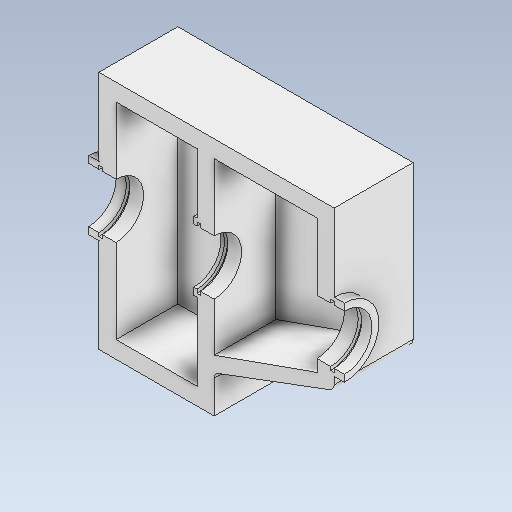
# Autodesk Inventor part: zmotorblockleft-half
Saved by Autodesk Inventor 2020 (Build 240168000, 168)
## iProperties
Created: 2020-11-21
Part Number: zmotorblockleft-half
Material: ABS Plastic
Document SubType Name: Modeling
Designer: AOB
Mass: 48.551 g
Surface Area: 203.359 cm^2
Volume: 45.8029 cm^3
Density: 1.06 g/cm^3
Appearance: Smooth - White
Author: AOB
Autodesk Inventor part; units mm, degrees
ref_plane "YZ Plane" through (0, 0, 0) normal (1, 0, 0) x (0, 1, 0)
sketch "Sketch1" plane through (0, 0, 0) normal (0, 0, 1) x (1, 0, 0)
  line L0 (16.1624, 3.9921) -> (16.1624, 53.6188)
  line L1 (16.0624, -11.3812) -> (-17.438, -11.3812)
  line L2 (-17.438, 58.6188) -> (48.5624, 58.6188)
  line L3 (-17.438, 58.6188) -> (-17.438, -11.3812)
  line L4 (-12.438, 53.6188) -> (-12.438, -6.3812)
  line L5 (11.1624, 53.6188) -> (11.1624, -6.3812)
  line L6 (43.5624, 53.6188) -> (46.1624, 53.6188)
  line L7 (11.1624, 53.6188) -> (-12.438, 53.6188)
  line L8 (-12.438, -6.3812) -> (11.1624, -6.3812)
  line L9 (18.7626, 0.4857) -> (43.5624, 9.7508)
  line L10 (16.1624, -1.8735) -> (16.1624, -11.3812)
  arc A0 (17.4625, 0) -> (16.1624, -1.8735) centre (18.1624, -1.8735) ccw
  line L11 (16.1624, -11.3812) -> (16.0624, -11.3812)
  line L12 (16.1624, 53.6188) -> (43.5624, 53.6188)
  line L13 (46.1624, 53.6188) -> (46.1624, 14.6188)
  line L14 (46.1624, 10.7222) -> (43.5624, 9.7508)
  line L15 (51.1624, 32.1705) -> (51.1624, 58.6188)
  line L16 (51.1624, 58.6188) -> (48.5624, 58.6188)
  line L17 (51.1624, 32.1705) -> (51.1624, 13.978)
  arc A1 (49.8624, 12.1045) -> (51.1624, 13.978) centre (49.1624, 13.978) ccw
  line L18 (46.1624, 14.6188) -> (16.1624, 3.9921)
  line L19 (17.4625, 0) -> (49.8624, 12.1045)
  point P0 (49.8624, 12.1045)
  point P1 (51.1624, 13.978)
  point P2 (-16.4376, 58.6188)
  point P3 (-16.4376, -11.3812)
  point P4 (16.1624, -1.8735)
  point P5 (17.4625, 0)
  point P6 (18.7626, 0.4857)
  point P7 (46.1624, 10.7222)
  point P8 (-11.4376, -6.3812)
  point P9 (-11.4376, 53.6188)
  constraints: 40 end point, 4 point on circle, 2 centre point
extrude "Extrusion5" add sketch "Sketch1" along normal blind 41 contours L1 L3 L2 L16 L15 L17 A1 L19 L14 L9 A0 L10 L11 | L7 L5 L8 L4
sketch "Sketch7" plane through (0, 0, 0) normal (0, 0, -1) x (-1, 0, 0)
  line L0 (17.438, 58.6188) -> (17.438, -11.3812)
  line L1 (-16.1624, -11.3812) -> (-16.1624, -1.8735) projected
  line L2 (17.438, -11.3812) -> (-16.1624, -11.3812)
  line L3 (-16.1624, -11.3812) -> (-16.1624, 0.8571)
  line L4 (-51.1624, 58.6188) -> (17.438, 58.6188) projected
  line L5 (17.438, 58.6188) -> (-51.1624, 58.6188)
  arc A0 (-51.1624, 13.978) -> (-49.8624, 12.1045) centre (-49.1624, 13.978) ccw projected
  line L6 (-51.1624, 58.6188) -> (-51.1624, 13.978)
  line L7 (-17.4625, 0) -> (-49.8624, 12.1045) projected
  line L8 (-49.8624, 12.1045) -> (-17.4625, 0)
  arc A1 (-16.1624, -1.8735) -> (-17.4625, 0) centre (-18.1624, -1.8735) ccw
  arc A2 (-51.1624, 13.978) -> (-49.8624, 12.1045) centre (-49.1624, 13.978) ccw
  point P0 (0, 0)
  point P1 (16.4376, 58.6188)
  point P2 (-16.1624, -1.8735)
  constraints: 12 end point, 4 point on circle, 3 perpendicular, 2 centre point, 2 point on line, 1 coincident, 1 collinear, 1 horizontal, 1 tangent
extrude "Extrusion6" add sketch "Sketch7" along normal blind 5
ref_plane "Work Plane11" through (0, 0, 18) normal (0, 0, 1) x (1, 0, 0)
sketch "Sketch10" plane through (51.1624, 13.978, 41) normal (1, 0, 0) x (0, 0, -1)
  circle A0 centre (23, 12.1408) radius 9
  circle A1 centre (23, 12.1408) radius 10
  circle A2 centre (23, 12.1408) radius 8
  dimension "d54" = 18
  dimension "d57" = 20
  dimension "d70" = 16
  constraints: 3 centre point, 3 coincident
  measures "d54" diameter of A0
  measures "d57" diameter of A1
  measures "d70" diameter of A2
extrude "Extrusion8" cut sketch "Sketch10" against normal blind 1 contours A0 | A2
extrude "Extrusion10" cut sketch "Sketch1" along normal through all contours L7 L5 L8 L4
hole "Hole4" at (51.1624, 26.1188, 18) direction (-1, 0, 0) diameter 16 end through all
extrude "Extrusion11" add sketch "Sketch10" along normal blind 3 contours A0 | A1
sketch "Sketch11" plane through (11.1624, -6.3812, 0) normal (-1, 0, 0) x (0, 0, 1)
  circle A0 centre (18, 32.5) radius 8 projected
  circle A1 centre (18, 32.5) radius 9 projected
  circle A2 centre (18, 32.5) radius 10 projected
  point P0 (0, 6.3812)
extrude "Extrusion12" cut sketch "Sketch11" against normal blind 1 contours A1
extrude "Extrusion13" add sketch "Sketch11" along normal blind 1 contours A1 | A2
sketch "Sketch12" plane through (-17.438, -11.3812, 41) normal (-1, 0, 0) x (0, 0, 1)
  circle A0 centre (-23, 37.5) radius 8 projected
  circle A1 centre (-23, 37.5) radius 9 projected
  circle A2 centre (-23, 37.5) radius 10 projected
  point P0 (-41, 11.3812)
extrude "Extrusion14" cut sketch "Sketch12" against normal blind 1 contours A1
extrude "Extrusion15" add sketch "Sketch12" along normal blind 3 contours A1 | A2
ref_plane "Work Plane13" through (0, 0, 18) normal (0, 0, -1) x (-1, 0, 0)
split "Split2" plane through (0, 0, 18) removes the side toward (0, 0, 1)
body "Solid2"
